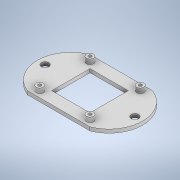
# Autodesk Inventor part: ephys_board_rack
Saved by Autodesk Inventor 2022 (Build 260153000, 153)
## iProperties
Created: 2021-09-06
Part Number: ephys_board_rack
Material: Generic
Document SubType Name: Modeling
Designer: dsdan
Density: 1 g/cm^3
Appearance: Default
Author: dsdan
Autodesk Inventor part; units mm, degrees
ref_plane "YZ Plane" through (0, 0, 0) normal (1, 0, 0) x (0, 1, 0)
ref_plane "XZ Plane" through (0, 0, 0) normal (0, 1, 0) x (-1, 0, 0)
ref_plane "XY Plane" through (0, 0, 0) normal (0, 0, 1) x (1, 0, 0)
sketch "Sketch1" plane through (0, 0, 0) normal (0, 1, 0) x (-1, 0, 0)
  line L0 (0, 0) -> (52.2, 0)
  line L1 (52.2, 0) -> (52.2, -52.2)
  line L2 (52.2, -52.2) -> (0, -52.2)
  line L3 (0, -52.2) -> (0, 0)
  circle A0 centre (47.1, -47.1) radius 1.3
  circle A1 centre (5.1, -5.1) radius 1.3
  circle A2 centre (5.1, -47.1) radius 1.3
  line L4 (0, 0) -> (52.2, -52.2) construction
  line L5 (52.2, 0) -> (0, -52.2) construction
  line L6 (5.1, -5.1) -> (47.1, -47.1) construction
  circle A3 centre (47.1, -5.1) radius 1.3
  circle A4 centre (63.6, -26.1) radius 3.1
  circle A5 centre (-11.4, -26.1) radius 3.1
  arc A6 (52.2, -52.2) -> (52.2, 0) centre (42.0615, -26.1) ccw
  arc A7 (0, 0) -> (0, -52.2) centre (10.1385, -26.1) ccw
  line L7 (10.1, -10.1) -> (10.1, -42.1)
  line L8 (10.1, -42.1) -> (42.1, -42.1)
  line L9 (42.1, -42.1) -> (42.1, -10.1)
  line L10 (42.1, -10.1) -> (10.1, -10.1)
  line L11 (10.1, -10.1) -> (42.1, -42.1) construction
  line L12 (10.1, -42.1) -> (42.1, -10.1) construction
  point P0 (26.1, -26.1)
  point P1 (26.1, -26.1)
  dimension "d1" = 42
  dimension "d2" = 42
  dimension "d3" = 2.6
  dimension "d4" = 2.6
  dimension "d5" = 2.6
  dimension "d18" = 52.2
  dimension "d19" = 52.2
  dimension "d24" = 2.6
  dimension "d26" = 6.2
  dimension "d27" = 6.2
  dimension "d28" = 75
  dimension "d29" = 37.5
  dimension "d30" = 28
  dimension "d31" = 28
  dimension "d32" = 32
  dimension "d33" = 32
  constraints: 26 end point, 8 centre point, 5 midpoint, 4 horizontal alignment, 4 parallel, 4 point on circle, 2 perpendicular, 2 vertical alignment, 1 horizontal, 1 vertical
  measures "d1" distance of A2.centre L6.start
  measures "d2" distance of L6.end A2.centre
  measures "d3" diameter of A0
  measures "d4" diameter of A2
  measures "d5" diameter of A1
  measures "d18" distance of L0.end L1.end
  measures "d19" distance of L1.end L2.end
  measures "d24" diameter of A3
  measures "d26" diameter of A4
  measures "d27" diameter of A5
  measures "d28" distance of A5.centre A4.centre
  measures "d29" distance of point (26.1, -26.1) A5.centre
  measures "d30" radius of A6
  measures "d31" radius of A7
  measures "d32" distance of L8.end L9.end
  measures "d33" distance between parallel lines of L7 L9
extrude "Extrusion1" add sketch "Sketch1" along normal blind 3
sketch "Sketch2" plane through (0, 3, 0) normal (0, 1, 0) x (1, 0, 0)
  circle A0 centre (-5.1, 5.1) radius 1.3 projected
  circle A1 centre (-5.1, 5.1) radius 3
  circle A2 centre (-5.1, 47.1) radius 1.3 projected
  circle A3 centre (-5.1, 47.1) radius 3
  circle A4 centre (-47.1, 47.1) radius 1.3 projected
  circle A5 centre (-47.1, 47.1) radius 3
  circle A6 centre (-47.1, 5.1) radius 1.3 projected
  circle A7 centre (-47.1, 5.1) radius 3
  point P0 (0, 0)
  dimension "d12" = 6
  dimension "d13" = 6
  dimension "d14" = 6
  dimension "d25" = 6
  constraints: 4 centre point, 4 coincident
  measures "d12" diameter of A5
  measures "d13" diameter of A1
  measures "d14" diameter of A3
  measures "d25" diameter of A7
extrude "Extrusion2" add sketch "Sketch2" along normal blind 4
equation "\"d4\" = d3"
equation "\"d5\" = d3"
equation "\"d19\" = d18"
equation "\"d24\" = d3"
equation "\"d27\" = d26"
equation "\"d29\" = 0.5 * d28"
equation "\"d33\" = d32"
equation "\"d13\" = d12"
equation "\"d14\" = d12"
equation "\"d25\" = d12"
equation "\"d7\" = d8"
equation "\"d8\" = 3"
body "Solid1"
